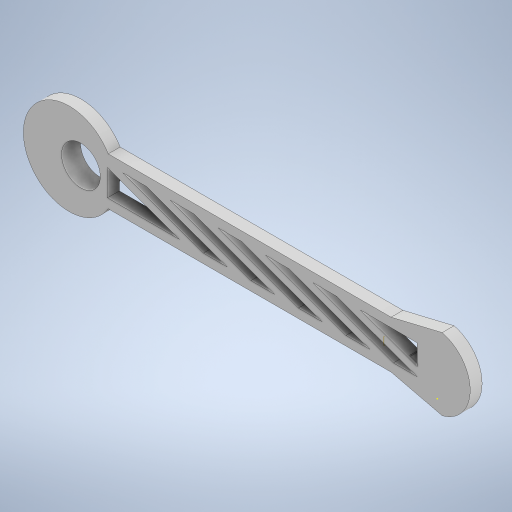
# Autodesk Inventor part: arm_v3
Saved by Autodesk Inventor 2024.3 (Build 283343000, 343)
## iProperties
Created: 2024-07-19
Part Number: arm_v3
Material: Ogólny
Document SubType Name: Modeling
Designer: User
Density: 1 g/cm^3
Appearance: Domyślna
Mass: 14.6731 g
Surface Area: 114.257 cm^2
Volume: 14.6731 cm^3
Author: User
Autodesk Inventor part; units mm, degrees
ref_plane "YZ Plane" through (0, 0, 0) normal (1, 0, 0) x (0, 1, 0)
ref_plane "XZ Plane" through (0, 0, 0) normal (0, 1, 0) x (-1, 0, 0)
sketch "Szkic1" plane through (0, 0, 0) normal (0, 1, 0) x (-1, 0, 0)
  line L0 (0, 0) -> (150, 0)
  line L1 (150, 0) -> (150, -5)
  line L2 (150, -5) -> (0, -5)
  line L3 (0, -5) -> (0, 0)
  dimension "d0" = 150
  dimension "d1" = 5
  constraints: 8 end point, 2 parallel, 1 horizontal, 1 perpendicular
  measures "d0" distance of L1.end L2.end
  measures "d1" distance of L0.end L1.end
extrude "Wyciągnięcie proste1" add sketch "Szkic1" along normal blind 20
sketch "Szkic2" plane through (0, 0, -5) normal (0, 0, -1) x (-1, 0, 0)
  line L0 (0, 0) -> (0, 20) projected
  circle A0 centre (0, 10) radius 2.95
  line L1 (0, 20) -> (-2, 20)
  line L2 (0, 0) -> (-2, 0)
  arc A1 (-2, 20) -> (-2, 0) centre (9.1803, 10) ccw
  line L3 (0, 10) -> (150, 10)
  line L4 (150, 10) -> (138.5, 10)
  line L5 (138.5, 10) -> (170.9, 10)
  line L6 (150, 0) -> (150, 20) projected
  line L7 (138.5, 10) -> (170.9, 10) construction
  line L8 (138.5, 10) -> (170.9, 10)
  line L9 (170.9, 10) -> (170.9, 16.16)
  line L10 (170.9, 16.16) -> (138.5, 16.16)
  line L11 (138.5, 16.16) -> (138.5, 10)
  line L12 (138.5, 10) -> (170.9, 10)
  line L13 (170.9, 10) -> (170.9, 3.84)
  line L14 (170.9, 3.84) -> (138.5, 3.84)
  line L15 (138.5, 3.84) -> (138.5, 10)
  line L16 (0, 0) -> (150, 0) projected
  line L17 (0, 20) -> (150, 20) projected
  arc A2 (138.5, 0) -> (138.5, 20) centre (154.9429, 10) ccw
  point P0 (150, 3.84)
  point P1 (150, 16.16)
  point P2 (0, 7.05)
  point P3 (0, 12.95)
  dimension "d4" = 5.9
  dimension "d5" = 2
  dimension "d6" = 2
  dimension "d7" = 15
  dimension "d8" = 150
  dimension "d9" = 11.5
  dimension "d10" = 32.4
  dimension "d11" = 0
  dimension "d12" = 6.16
  dimension "d13" = 6.16
  constraints: 28 end point, 6 horizontal, 4 parallel, 4 point on circle, 4 point on line, 3 centre point, 3 perpendicular, 1 collinear, 1 midpoint
  measures "d4" diameter of A0
  measures "d5" distance of L0.end L1.end
  measures "d6" distance of L0.start L2.end
  measures "d7" radius of A1
  measures "d8" distance of L3.start L3.end
  measures "d9" distance of L3.end L4.end
  measures "d10" distance of L4.end L5.end
  measures "d11" distance between parallel lines of L5 L7
  measures "d12" distance of L9.end L8.end
  measures "d13" distance of L12.end L13.end
extrude "Wyciągnięcie proste2" add sketch "Szkic2" against normal blind 5 contours L2 A1 L1 L0 A0 | L16 L6 L14 L13 L9 L10 L17 A2
sketch "Szkic3" plane through (2, 20, -5) normal (0, 0, -1) x (-1, 0, 0)
  arc A0 (2, -7.05) -> (2, -12.95) centre (2, -10) ccw projected
  circle A1 centre (2, -10) radius 2.95
  line L0 (152, -16.16) -> (152, -3.84) projected
  line L1 (152, -16.16) -> (150.5, -16.16)
  line L2 (150.5, -16.16) -> (150.5, -3.84)
  line L3 (150.5, -3.84) -> (152, -3.84)
  line L4 (140.5, -16.16) -> (10.5, -16.16)
  line L5 (10.5, -16.16) -> (10.5, -3.84)
  line L6 (10.5, -3.84) -> (140.5, -3.84)
  line L7 (140.5, -3.84) -> (140.5, -16.16)
  line L8 (150.5, -16.16) -> (150.3, -16.16)
  line L9 (150.3, -16.16) -> (150.3, -3.84)
  line L10 (150.3, -3.84) -> (150.5, -3.84)
  line L11 (152, -16.16) -> (140.5, -16.16)
  line L12 (140.5, -16.16) -> (140.5, -3.84)
  line L13 (140.5, -3.84) -> (152, -3.84)
  line L14 (152, -3.84) -> (152, -16.16)
  point P0 (2, -20)
  dimension "d16" = 1.5
  dimension "d17" = 130
  dimension "d18" = 12.32
  dimension "d21" = 0.2
  dimension "d24" = 11.5
  constraints: 28 end point, 5 perpendicular, 4 horizontal, 4 parallel, 1 centre point, 1 coincident, 1 vertical
  measures "d16" distance of L0.start L1.end
  measures "d17" distance of L5.end L6.end
  measures "d18" distance of L4.end L5.end
  measures "d21" distance of L1.end L8.end
  measures "d24" distance of L6.end L13.end
extrude "Wyciągnięcie proste3" cut sketch "Szkic3" against normal through all
sketch "Szkic5" plane through (2, 20, -5) normal (0, 0, -1) x (-1, 0, 0)
  circle A0 centre (2, -10) radius 2.95 projected
  line L0 (2, -10) -> (152, -10)
  line L1 (2, -10) -> (152, -10) construction
  circle A1 centre (152, -10) radius 5.0551
  line L2 (152, -10) -> (145.8, -10)
  line L3 (145.8, -10) -> (145.8, -3.84)
  line L4 (10.5, -3.84) -> (172.9, -3.84) projected
  line L5 (145.8, -3.84) -> (140.8, -3.84)
  line L6 (140.8, -3.84) -> (140.8, -16.16)
  line L7 (172.9, -16.16) -> (10.5, -16.16) projected
  line L8 (145.8, -10) -> (145.8, -16.16)
  line L9 (145.8, -16.16) -> (140.8, -16.16)
  line L10 (10.5, -16.16) -> (10.5, -3.84) projected
  line L11 (10.5, -16.16) -> (44.3489, -3.84)
  line L12 (10.5, -16.16) -> (46.5213, -16.16) construction
  line L13 (44.3489, -3.84) -> (54.3489, -3.84)
  line L14 (10.5, -16.16) -> (20.5, -16.16)
  line L15 (20.5, -16.16) -> (54.3489, -3.84)
  line L16 (20.5, -16.16) -> (30.5, -16.16)
  line L17 (54.3489, -3.84) -> (64.3489, -3.84)
  line L18 (64.3489, -3.84) -> (30.5, -16.16)
  line L19 (44.3489, -3.84) -> (34.3489, -3.84)
  line L20 (10.5, -16.16) -> (0.5, -16.16)
  line L21 (0.5, -16.16) -> (34.3489, -3.84)
  line L22 (40.5, -16.16) -> (74.3489, -3.84)
  line L23 (50.5, -16.16) -> (84.3489, -3.84)
  line L24 (94.3489, -3.84) -> (60.5, -16.16)
  line L25 (30.5, -16.16) -> (64.3489, -3.84)
  line L26 (70.5, -16.16) -> (104.3489, -3.84)
  line L27 (80.5, -16.16) -> (114.3489, -3.84)
  line L28 (124.3489, -3.84) -> (90.5, -16.16)
  line L29 (60.5, -16.16) -> (94.3489, -3.84)
  line L30 (100.5, -16.16) -> (134.3489, -3.84)
  line L31 (110.5, -16.16) -> (144.3489, -3.84)
  line L32 (90.5, -16.16) -> (124.3489, -3.84)
  point P0 (2, -20)
  point P1 (10.5, -12.5203)
  point P2 (60.5, -16.16)
  point P3 (140.8, -5.1317)
  dimension "d25" = 150
  dimension "d26" = 0
  dimension "d27" = 6.2
  dimension "d28" = 5
  dimension "d29" = 20
  dimension "d30" = 10
  dimension "d31" = 10
  dimension "d32" = 10
  dimension "d33" = 10
  dimension "d34" = 10
  dimension "d35" = 10
  dimension "d36" = 10
  dimension "d37" = 10
  dimension "d38" = 10
  dimension "d39" = 10
  dimension "d40" = 10
  dimension "d41" = 10
  dimension "d42" = 10
  dimension "d43" = 10
  dimension "d44" = 10
  dimension "d45" = 10
  dimension "d46" = 10
  dimension "d47" = 10
  dimension "d48" = 10
  dimension "d49" = 10
  dimension "d52" = 10
  dimension "d53" = 10
  constraints: 60 end point, 10 point on line, 4 horizontal, 2 equal length, 2 perpendicular, 2 vertical, 1 centre point, 1 coincident
  measures "d25" distance of L0.start L0.end
  measures "d26" distance between parallel lines of L0 L1
  measures "d27" distance of L2.start L2.end
  measures "d28" distance of L3.end L5.end
  measures "d29" angle of L12 L11
  measures "d30" distance of L11.end L13.end
  measures "d31" distance of L7.end L14.end
  measures "d32" distance of L14.end L16.end
  measures "d33" distance of L13.end L17.end
  measures "d34" distance of L11.end L19.end
  measures "d35" distance of L7.end L20.end
  measures "d36" distance of L22.end L23.end
  measures "d37" distance of L22.start L23.start
  measures "d38" distance of L23.start L24.end
  measures "d39" distance of L23.end L24.start
  measures "d40" distance of L22.end L25.end
  measures "d41" distance of L22.start L25.start
  measures "d42" distance of L26.end L27.end
  measures "d43" distance of L26.start L27.start
  measures "d44" distance of L27.start L28.end
  measures "d45" distance of L27.end L28.start
  measures "d46" distance of L26.end L29.end
  measures "d47" distance of L26.start L29.start
  measures "d48" distance of L30.end L31.end
  measures "d49" distance of L30.start L31.start
  measures "d52" distance of L30.end L32.end
  measures "d53" distance of L30.start L32.start
extrude "Wyciągnięcie proste4" add sketch "Szkic5" against normal blind 5 contours L21 L4 L11 L0 | L0 L11 L10 L21 | L15 L4 L18 L0 | L0 L18 L7 L15 | L22 L4 L23 L0 | L0 L23 L7 L22 | L24 L4 L26 L0 | L0 L26 L7 L24 | L27 L4 L28 L0 | L0 L28 L7 L27 | L30 L4 L6 L31 L0 | L0 L31 L7 L30 | L6 L31 L4 L3 L0 | L0 L8 L7 L6 | L6 L4 L31
sketch "Szkic6" plane through (-138.5, 0, 0) normal (0, 0, 1) x (1, 0, 0)
  circle A0 centre (138.5, 10) radius 2.95 projected
  circle A1 centre (138.5, 10) radius 2.85
  circle A2 centre (138.5, 10) radius 2.95
  point P0 (138.5, 0)
  dimension "d56" = 5.7
  constraints: 2 centre point, 2 coincident
  measures "d56" diameter of A1
extrude "Wyciągnięcie proste5" add sketch "Szkic6" against normal blind 5
ref_plane "Płaszczyzna konstrukcyjna1" through (-138.5, 0, -1) normal (0, 0, 1) x (1, 0, 0)
sketch "Szkic7" plane through (-138.5, 0, -1) normal (0, 0, 1) x (1, 0, 0)
  circle A0 centre (138.5, 10) radius 2.85 projected
  circle A1 centre (138.5, 10) radius 1.25
  circle A2 centre (138.5, 10) radius 2.85
  point P0 (138.5, 0)
  dimension "d60" = 2.5
  constraints: 2 centre point, 2 coincident
  measures "d60" diameter of A1
extrude "Wyciągnięcie proste6" add sketch "Szkic7" against normal blind 1
sketch "Szkic8" plane through (-138.5, 0, 0) normal (0, 0, 1) x (1, 0, 0)
  point P0 (138.5, 0)
sketch "Szkic9" plane through (-138.5, 0, 0) normal (0, 0, 1) x (1, 0, 0)
  circle A0 centre (138.5, 10) radius 1.25 projected
  line L0 (138.5, 10) -> (-11.5, 10)
  line L1 (138.5, 10) -> (288.5, 10) construction
  circle A1 centre (-11.5, 10) radius 8.15
  point P0 (138.5, 0)
  dimension "d63" = 150
  dimension "d64" = 180
  dimension "d65" = 16.3
  constraints: 4 end point, 2 horizontal, 1 centre point, 1 coincident, 1 collinear
  measures "d63" distance of L0.start L0.end
  measures "d64" angle of L0 L1
  measures "d65" diameter of A1
extrude "Wyciągnięcie proste7" cut sketch "Szkic9" against normal through all contours A1
sketch "Szkic10" plane through (-138.5, 0, 0) normal (0, 0, 1) x (1, 0, 0)
  arc A0 (-5.3, 4.7102) -> (-5.3, 15.2898) centre (-11.5, 10) ccw projected
  circle A1 centre (-11.5, 10) radius 8.15
  line L0 (-32.5164, 20) -> (-2.9538, 20)
  line L1 (-2.9538, 20) -> (-2.9538, 1.85)
  line L2 (-2.9538, 1.85) -> (-32.5164, 1.85)
  line L3 (-32.5164, 1.85) -> (-32.5164, 20)
  point P0 (138.5, 0)
  point P1 (-11.5, 1.85)
  point P2 (-5.3, 15.2898)
  constraints: 8 end point, 2 parallel, 1 centre point, 1 coincident, 1 horizontal, 1 perpendicular
extrude "Wyciągnięcie proste8" add sketch "Szkic10" against normal blind 5
sketch "Szkic11" plane through (2, 20, -5) normal (0, 0, -1) x (-1, 0, 0)
  circle A0 centre (152, -10) radius 8.15 projected
  circle A1 centre (152, -10) radius 8.15
  circle A2 centre (152, -10) radius 10
  point P0 (2, -20)
  dimension "d70" = 20
  constraints: 2 centre point, 2 coincident
  measures "d70" diameter of A2
extrude "Wyciągnięcie proste9" add sketch "Szkic11" along normal blind 3
sketch "Szkic12" plane through (2, 20, -5) normal (0, 0, -1) x (-1, 0, 0)
  circle A0 centre (2, -10) radius 1.25 projected
  circle A1 centre (2, -10) radius 5.2
  arc A2 (0, 0) -> (0, -20) centre (11.1803, -10) ccw projected
  line L0 (2, -10) -> (14.7, -10)
  line L1 (2, -10) -> (2, 2.7)
  line L2 (2, -10) -> (-10.7, -10)
  line L3 (2, -10) -> (2, -22.7)
  line L4 (2, -15.2) -> (6, -15.2)
  line L5 (6, -15.2) -> (2, -15.2)
  line L6 (2, -15.2) -> (-2, -15.2)
  line L7 (7.2, -10) -> (7.2, -6)
  line L8 (7.2, -10) -> (7.2, -14)
  line L9 (2, -4.8) -> (-2, -4.8)
  line L10 (2, -4.8) -> (6, -4.8)
  line L11 (-3.2, -10) -> (-3.2, -14)
  line L12 (-3.2, -10) -> (-3.2, -6)
  line L13 (2, -22.7) -> (3.5, -22.7)
  line L14 (3.5, -22.7) -> (2, -22.7)
  line L15 (2, -22.7) -> (0.5, -22.7)
  line L16 (3.5, -22.7) -> (6, -15.2)
  line L17 (0.5, -22.7) -> (-2, -15.2)
  line L18 (14.7, -8.5) -> (7.2, -6)
  line L19 (14.7, -11.5) -> (7.2, -14)
  line L20 (14.7, -8.5) -> (14.7, -10)
  line L21 (0.5, 2.7) -> (-2, -4.8)
  line L22 (3.5, 2.7) -> (6, -4.8)
  line L23 (0.5, 2.7) -> (2, 2.7)
  line L24 (-10.7, -11.5) -> (-3.2, -14)
  line L25 (-10.7, -8.5) -> (-3.2, -6)
  line L26 (-10.7, -11.5) -> (-10.7, -10)
  line L27 (-10.7, -11.5) -> (-10.7, -8.5)
  line L28 (14.7, -11.5) -> (14.7, -8.5)
  line L29 (3.5, 2.7) -> (0.5, 2.7)
  arc A3 (7.2, -6) -> (6, -4.8) centre (5.3194, -6.6806) ccw
  arc A4 (-2, -4.8) -> (-3.2, -6) centre (-1.3194, -6.6806) ccw
  arc A5 (-3.2, -14) -> (-2, -15.2) centre (-1.3194, -13.3194) ccw
  arc A6 (6, -15.2) -> (7.2, -14) centre (5.3194, -13.3194) ccw
  point P0 (2, -20)
  dimension "d73" = 10.4
  dimension "d75" = 12.7
  dimension "d76" = 12.7
  dimension "d77" = 12.7
  dimension "d78" = 12.7
  dimension "d79" = 4
  dimension "d80" = 4
  dimension "d83" = 360
  dimension "d85" = 1.5
  dimension "d86" = 1.5
  dimension "d89" = 360
  dimension "d91" = 2
  dimension "d92" = 2
  dimension "d93" = 2
  dimension "d94" = 2
  constraints: 60 end point, 8 point on circle, 7 horizontal, 5 point on line, 4 centre point, 4 collinear, 3 vertical, 1 coincident, 1 perpendicular, 1 vertical alignment, 56 other
  measures "d75" distance of L0.start L0.end
  measures "d76" distance of L0.start L1.end
  measures "d77" distance of L0.start L2.end
  measures "d78" distance of L0.start L3.end
  measures "d79" distance of L4.start L4.end
  measures "d80" distance of L4.start L6.end
  measures "d85" distance of L3.end L13.end
  measures "d86" distance of L3.end L15.end
  measures "d91" radius of A3
  measures "d92" radius of A4
  measures "d93" radius of A5
  measures "d94" radius of A6
sketch "Szkic13" plane through (2, 20, -5) normal (0, 0, -1) x (-1, 0, 0)
  line L0 (140.5, 0) -> (0, 0) projected
  line L1 (21.4996, 0) -> (0, 5.1324)
  arc A0 (0, 0) -> (0, -20) centre (11.1803, -10) ccw projected
  line L2 (-3.8197, -10) -> (24.797, -10)
  line L3 (21.4996, -20) -> (0, -25.1324)
  arc A1 (0, 5.1324) -> (0, -25.1324) centre (3.8411, -10) ccw
  line L4 (21.4996, 0) -> (21.4996, -20)
  line L5 (140.5, -20) -> (0, -20) projected
  point P0 (2, -20)
  constraints: 8 end point, 3 point on circle, 2 symmetric about line, 1 centre point, 1 horizontal, 1 perpendicular, 1 point on line
extrude "Wyciągnięcie proste10" add sketch "Szkic13" against normal blind 5 contours L0 A0 L5 L3 A1 L1
extrude "Wyciągnięcie proste11" cut sketch "Szkic12" against normal blind 4 contours L0 L1 A0 | L0 A1 L3 A0 | A0 L3 L0 | A0 L1 A1 L0 | L1 L2 A0 | A0 L2 A1 L1 | L3 A1 L2 A0 | A0 L2 L3 | L8 A6 L4 A1 | L7 L18 L20 L0 | A1 L10 A3 L7 | L0 L28 L19 L8 | L9 L21 L23 L1 | A1 L12 A4 L9 | L1 L29 L22 L10 | L6 A5 L11 A1 | L4 L16 L13 L3 | L3 L15 L17 L6 | L11 L24 A2 L2 | L2 A2 L25 L12 | L2 L27 L25 A2 | A2 L24 L26 L2
ref_plane "Płaszczyzna konstrukcyjna2" through (-22.3, 8.5, -5) normal (-1, 0, 0) x (0, 0, 1)
sketch "Szkic14" plane through (-154.9429, 10, 0) normal (0, 0, 1) x (1, 0, 0)
  circle A0 centre (154.9429, 0) radius 2.85 projected
  circle A1 centre (154.9429, 0) radius 2.85
  point P0 (154.9429, -10)
  constraints: 1 centre point, 1 coincident
extrude "Wyciągnięcie proste12" add sketch "Szkic14" against normal blind 1
